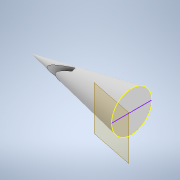
# Autodesk Inventor part: bishop
Saved by Autodesk Inventor 2021 (Build 250183000, 183)
## iProperties
Created: 2021-01-20
Part Number: bishop
Material: Generic
Document SubType Name: Modeling
Designer: Luke Kamols
Density: 1 g/cm^3
Appearance: Default
Author: Luke Kamols
Autodesk Inventor part; units mm, degrees
ref_plane "YZ Plane" through (0, 0, 0) normal (1, 0, 0) x (0, 1, 0)
ref_plane "XZ Plane" through (0, 0, 0) normal (0, 1, 0) x (-1, 0, 0)
ref_plane "XY Plane" through (0, 0, 0) normal (0, 0, 1) x (1, 0, 0)
sketch "Sketch1" plane through (0, 0, 0) normal (0, 1, 0) x (-1, 0, 0)
  line L0 (0, 0) -> (0, -10)
  line L1 (0, 0) -> (50, 0)
  line L2 (50, 0) -> (0, -10)
  dimension "d0" = 10
  dimension "d1" = 50
  constraints: 6 end point, 1 horizontal, 1 vertical
  measures "d0" distance of L0.start L0.end
  measures "d1" distance of L0.start L1.end
revolve "Revolution1" add sketch "Sketch1" angle 360 about axis through (0, 0, 0) along (-1, 0, 0)
sketch "Sketch2" plane through (0, 0, 0) normal (1, 0, 0) x (0, 0, -1)
  circle A0 centre (0, 0) radius 10 projected
  line L0 (-10, 0) -> (10, 0)
  circle A1 centre (0, 0) radius 10 projected
  constraints: 2 end point, 1 horizontal, 1 horizontal alignment, 1 point on circle, 1 other
ref_plane "Work Plane1" through (0, 0, 10) normal (-0.1961, 0, 0.9806) x (0, -1, 0)
sketch "Sketch3" plane through (0, 0, 0) normal (0, 1, 0) x (-1, 0, 0)
  line L0 (50, 0) -> (0, -10) projected
  line L1 (0, 10) -> (0, -10) projected
  line L2 (50, 0) -> (0, 10) projected
  line L3 (50, 0) -> (40.1942, 1.9612)
  line L4 (40.1942, 1.9612) -> (28.4272, -0.3922)
  line L5 (28.4272, -0.3922) -> (28.035, 1.5689)
  line L6 (28.035, 1.5689) -> (35.0952, 2.981)
  point P0 (0, 0)
  point P1 (50, 0)
  dimension "d3" = 10
  dimension "d4" = 12
  dimension "d6" = 2
  constraints: 8 end point, 2 point on line, 1 perpendicular
  measures "d3" distance of L2.start L3.end
  measures "d4" distance of L3.end L4.end
  measures "d6" distance of L4.end L5.end
extrude "Extrusion1" cut sketch "Sketch3" along normal mid plane 10 contours L4 L5 L6 L2
body "Solid1"
